stdRS22087 (Autodesk Fusion 360 design; units mm, degrees)
Autodesk Fusion 360 part; units mm, degrees
sketch "Esquisse1" plane through (0, 0, 0) normal (0, 0, 1) x (1, 0, 0)
  circle A0 centre (0, 0) radius 11
  circle A1 centre (0, 0) radius 4
  dimension "d59" = 22
  dimension "d60" = 8
  constraint coincident A0.centre A1.centre
  measures "d59" diameter of A0
  measures "d60" diameter of A1
extrude "Extrusion1" add sketch "Esquisse1" along normal blind 7
